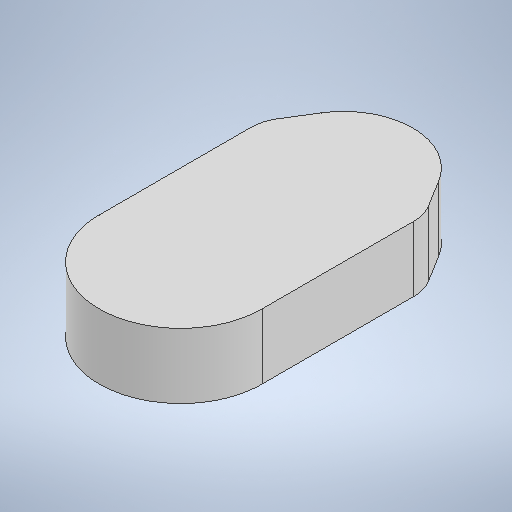
# Autodesk Inventor part: Servo_Shaft_select_V1
Saved by Autodesk Inventor 2025.3 (Build 293356000, 356)
## iProperties
Created: 2026-04-10
Part Number: Servo_Shaft_select_V1
Material: Generic
Document SubType Name: Modeling
Designer: kamal
Density: 1 g/cm^3
Appearance: Default
Mass: 5.65431 g
Surface Area: 27.7969 cm^2
Volume: 5.65431 cm^3
Author: kamal
Autodesk Inventor part; units mm, degrees
ref_plane "YZ Plane" through (0, 0, 0) normal (1, 0, 0) x (0, 1, 0)
ref_plane "XZ Plane" through (0, 0, 0) normal (0, 1, 0) x (-1, 0, 0)
ref_plane "XY Plane" through (0, 0, 0) normal (0, 0, 1) x (1, 0, 0)
sketch "Sketch1" plane through (0, 0, 0) normal (0, 1, 0) x (-1, 0, 0)
  arc A0 (-2.75, 2.1651) -> (2.75, 2.1651) centre (0, 0) ccw
  line L0 (-1.9, 14.1) -> (-2.75, 2.1651)
  line L1 (1.8987, 14.0987) -> (2.75, 2.1651)
  arc A1 (1.8987, 14.0987) -> (-1.9, 14.1) centre (-0.0007, 14.05) ccw
  circle A2 centre (0, 0) radius 0.5
  line L2 (0, 0) -> (0, -10) construction
  line L3 (0, 30) -> (0, 0) construction
  arc A3 (-7.6535, 3.6978) -> (7.6533, 3.6982) centre (0, 0) ccw
  line L4 (7.6533, 3.6982) -> (6.8916, 14.3762)
  arc A4 (6.8916, 14.3762) -> (-6.8928, 14.3783) centre (-0.0007, 14.05) ccw
  line L5 (-6.8928, 14.3783) -> (-7.6535, 3.6978)
  line L6 (10, 0) -> (-10, 0)
  line L7 (-10, 0) -> (-10, 30)
  line L8 (-10, 30) -> (10, 30)
  line L9 (10, 30) -> (10, 0)
  point P0 (-8.5, 0)
  point P1 (8.5, 0)
  dimension "d0" = 1
  dimension "d9" = 1.9
  dimension "d11" = 3.5
  dimension "d34" = 10
  dimension "d42" = 5
  dimension "d43" = 20
  dimension "d44" = 30
  constraints: 20 end point, 8 point on circle, 5 centre point, 2 perpendicular, 2 vertical, 1 coincident, 1 collinear, 1 concentric, 1 horizontal, 1 midpoint, 3 other
  measures "d0" diameter of A2
  measures "d9" radius of A1
  measures "d11" radius of A0
  measures "d34" distance of L2.start L2.end
  measures "d42" distance between parallel lines of L0 L5
  measures "d43" distance of L6.start L6.end
  measures "d44" distance of L6.end L7.end
extrude "Extrusion6" add sketch "Sketch1" along normal blind 8 contours A0 L6 A3 L5 A4 L4 L1 A1 L0 | A0 L6 A3 | L6 L7 L8 L9 A3 L4 A4 L5
sketch "Sketch7" plane through (0, 0, 0) normal (0, -1, 0) x (1, 0, 0)
  arc A0 (-8.5, 0) -> (8.5, 0) centre (0, 0) ccw projected
  line L0 (10, 30) -> (10, 0) projected
  line L1 (-10, 0) -> (-10, 30) projected
  line L2 (-10, 0) -> (-10, 30) projected
  line L3 (-10, 0) -> (-7.225, -4.4777)
  line L4 (10, 0) -> (7.225, -4.4777)
  line L5 (8.5, 0) -> (10, 0)
  line L6 (-8.5, 0) -> (-10, 0) projected
  line L7 (-8.5, 0) -> (-10, 0)
  constraints: 8 end point, 3 point on circle, 2 collinear, 2 tangent
extrude "Extrusion7" add sketch "Sketch7" against normal blind 8
fillet "Fillet1" radius 5 2 edges at (10, 4, 0) (-10, 4, 0)
sketch "Sketch8" plane through (0, 0, 0) normal (0, -1, 0) x (1, 0, 0)
  arc A0 (-10, 1.4237) -> (-9.25, -1.2102) centre (-5, 1.4237) ccw projected
  line L0 (-9.25, -1.2102) -> (-7.225, -4.4777) projected
  arc A1 (-7.225, -4.4777) -> (7.225, -4.4777) centre (0, 0) ccw projected
  line L1 (7.225, -4.4777) -> (9.25, -1.2102) projected
  arc A2 (9.25, -1.2102) -> (10, 1.4237) centre (5, 1.4237) ccw projected
  line L2 (10, 30) -> (10, 1.4237) projected
  line L3 (-10, 30) -> (10, 30) projected
  line L4 (-10, 1.4237) -> (-10, 30) projected
  arc A3 (-2.75, 2.1651) -> (2.75, 2.1651) centre (0, 0) ccw projected
  line L5 (-1.8987, 14.0987) -> (-2.75, 2.1651) projected
  arc A4 (1.9, 14.1) -> (-1.8987, 14.0987) centre (0.0007, 14.05) ccw projected
  line L6 (2.75, 2.1651) -> (1.9, 14.1) projected
  circle A5 centre (0, 20) radius 10
  line L7 (10, 30) -> (10, 1.4237) projected
  line L8 (-10, 30) -> (10, 30) projected
  point P0 (-10, 20)
  point P1 (0, 30)
  point P2 (10, 20)
  dimension "d50" = 20
  constraints: 2 tangent, 1 centre point
  measures "d50" diameter of A5
extrude "Extrusion8" cut sketch "Sketch8" against normal through all contours L4 L3 A5 | L3 L2 A5
sketch "Sketch9" plane through (0, 8, 0) normal (0, 1, 0) x (1, 0, 0)
  arc A0 (-10, -20) -> (10, -20) centre (0, -20) ccw projected
  line L0 (-10, -1.4237) -> (-10, -20) projected
  arc A1 (-9.25, 1.2102) -> (-10, -1.4237) centre (-5, -1.4237) ccw projected
  line L1 (-7.225, 4.4777) -> (-9.25, 1.2102) projected
  arc A2 (7.225, 4.4777) -> (-7.225, 4.4777) centre (0, 0) ccw projected
  line L2 (9.25, 1.2102) -> (7.225, 4.4777) projected
  arc A3 (10, -1.4237) -> (9.25, 1.2102) centre (5, -1.4237) ccw projected
  line L3 (10, -20) -> (10, -1.4237) projected
extrude "Extrusion9" add sketch "Sketch9" against normal blind 5
body "Solid2"
